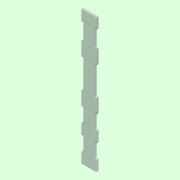
# Autodesk Inventor part: Left_wall
Saved by Autodesk Inventor 2015 (Build 190159000, 159)
## iProperties
Created: 2015-06-19
Part Number: Left_wall
Material: Generic
Document SubType Name: Modeling
Designer: Openlab
Density: 1 g/cm^3
Appearance: Polycarbonate - Clear
Author: Openlab
Autodesk Inventor part; units mm, degrees
ref_plane "YZ Plane" through (0, 0, 0) normal (1, 0, 0) x (0, 1, 0)
ref_plane "XZ Plane" through (0, 0, 0) normal (0, 1, 0) x (-1, 0, 0)
ref_plane "XY Plane" through (0, 0, 0) normal (0, 0, 1) x (1, 0, 0)
sketch "Sketch1" plane through (0, 0, 0) normal (0, 1, 0) x (-1, 0, 0)
  line L0 (21, -15) -> (18.25, -15)
  line L1 (21, -38) -> (18.25, -38)
  line L2 (21, -138) -> (18.25, -138)
  line L3 (21, -58) -> (18.25, -58)
  line L4 (21, -118) -> (18.25, -118)
  line L5 (21, -98) -> (18.25, -98)
  line L6 (2.75, -58) -> (0, -58)
  line L7 (2.75, -98) -> (0, -98)
  line L8 (2.75, -118) -> (0, -118)
  line L9 (2.75, -138) -> (0, -138)
  line L10 (2.75, -38) -> (0, -38)
  line L11 (2.75, -15) -> (0, -15)
  line L12 (21, -153) -> (21, -138)
  line L13 (21, -118) -> (21, -98)
  line L14 (21, -58) -> (21, -38)
  line L15 (21, -15) -> (21, 0)
  line L16 (0, -153) -> (0, -138)
  line L17 (0, -118) -> (0, -98)
  line L18 (0, -58) -> (0, -38)
  line L19 (0, -15) -> (0, 0)
  line L20 (18.25, -138) -> (18.25, -118)
  line L21 (18.25, -98) -> (18.25, -58)
  line L22 (18.25, -38) -> (18.25, -15)
  line L23 (2.75, -138) -> (2.75, -118)
  line L24 (2.75, -98) -> (2.75, -58)
  line L25 (2.75, -38) -> (2.75, -15)
  line L26 (21, -58) -> (21, -38) construction
  line L27 (2.75, -173) -> (2.75, -153)
  line L28 (21, 0) -> (0, 0)
  line L29 (21, -153) -> (18.25, -153)
  line L30 (2.75, -153) -> (0, -153)
  line L31 (18.25, -153) -> (18.25, -173)
  line L32 (18.25, -173) -> (21, -173)
  line L33 (21, -173) -> (21, -188)
  line L34 (21, -188) -> (0, -188)
  line L35 (0, -188) -> (0, -173)
  line L36 (0, -173) -> (2.75, -173)
  dimension "d7" = 23
  dimension "d8" = 20
  dimension "d9" = 40
  dimension "d10" = 20
  dimension "d11" = 20
  dimension "d28" = 15.5
  dimension "d31" = 2.75
  dimension "d38" = 15
  dimension "d39" = 20
  dimension "d40" = 15
  dimension "d41" = 15
  constraints: 75 end point, 29 collinear, 6 perpendicular, 4 parallel, 3 vertical, 2 point on line
  measures "d7" distance between parallel lines of L1 L0
  measures "d8" distance between parallel lines of L3 L1
  measures "d9" distance between parallel lines of L5 L3
  measures "d10" distance between parallel lines of L4 L5
  measures "d11" distance between parallel lines of L2 L4
  measures "d28" distance between parallel lines of L23 L20
  measures "d31" distance between parallel lines of L22 L15
  measures "d38" distance of L12.start L2.start
  measures "d39" distance of L29.end L31.end
  measures "d40" distance of L32.end L33.end
  measures "d41" distance between parallel lines of L0 L28
extrude "Extrusion3" add sketch "Sketch1" along normal blind 3
body "Solid3"
